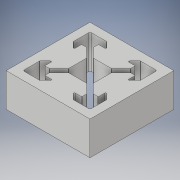
# Autodesk Inventor part: StepperMount
Saved by Autodesk Inventor 2019.4 (Build 234330000, 330)
## iProperties
Created: 2020-12-22
Part Number: StepperMount
Material: Generic
Document SubType Name: Modeling
Designer: Jorian Brusind
Density: 1 g/cm^3
Appearance: Default
Author: Jorian Brusind
Autodesk Inventor part; units mm, degrees
ref_plane "YZ Plane" through (0, 0, 0) normal (1, 0, 0) x (0, 1, 0)
ref_plane "XZ Plane" through (0, 0, 0) normal (0, 1, 0) x (-1, 0, 0)
ref_plane "XY Plane" through (0, 0, 0) normal (0, 0, 1) x (1, 0, 0)
sketch "2020 profile" plane through (0, 0, 0) normal (0, 0, 1) x (1, 0, 0)
  line L0 (8.75, -15.1376) -> (8.75, -9.8624)
  line L1 (2.5, -7.4482) -> (2.5, -3)
  line L2 (4.0732, -9.0732) -> (2.5366, -7.5366)
  line L3 (4.5, -7.125) -> (4.5, -8.8964)
  line L4 (5.8876, -7) -> (4.625, -7)
  line L5 (7, -4.625) -> (7, -5.8876)
  line L6 (7.0366, -5.976) -> (9.774, -8.7134)
  line L7 (8.8964, -4.5) -> (7.125, -4.5)
  line L8 (7.5366, -2.5366) -> (9.0732, -4.0732)
  line L9 (3, -2.5) -> (7.4482, -2.5)
  line L10 (17.5518, -2.5) -> (22, -2.5)
  arc A0 (22.5, -3) -> (22, -2.5) centre (22, -3) ccw
  line L11 (22.5, -3) -> (22.5, -7.4482)
  line L12 (22.4634, -7.5366) -> (20.9268, -9.0732)
  line L13 (20.5, -8.8964) -> (20.5, -7.125)
  line L14 (20.375, -7) -> (19.1124, -7)
  line L15 (18, -5.8876) -> (18, -4.625)
  line L16 (17.875, -4.5) -> (16.1036, -4.5)
  line L17 (15.226, -8.7134) -> (17.9634, -5.976)
  line L18 (19.024, -7.0366) -> (16.2866, -9.774)
  line L19 (16.25, -9.8624) -> (16.25, -15.1376)
  line L20 (16.2866, -15.226) -> (19.024, -17.9634)
  line L21 (19.1124, -18) -> (20.375, -18)
  arc A1 (19.024, -17.9634) -> (19.1124, -18) centre (19.1124, -17.875) ccw
  arc A2 (20.375, -18) -> (20.5, -17.875) centre (20.375, -17.875) ccw
  line L22 (20.5, -17.875) -> (20.5, -16.1036)
  arc A3 (20.9268, -15.9268) -> (20.5, -16.1036) centre (20.75, -16.1036) ccw
  line L23 (20.9268, -15.9268) -> (22.4634, -17.4634)
  arc A4 (22.5, -17.5518) -> (22.4634, -17.4634) centre (22.375, -17.5518) ccw
  line L24 (22.5, -17.5518) -> (22.5, -22)
  line L25 (22, -22.5) -> (17.5518, -22.5)
  line L26 (17.4634, -22.4634) -> (15.9268, -20.9268)
  arc A5 (16.1036, -20.5) -> (15.9268, -20.9268) centre (16.1036, -20.75) ccw
  line L27 (16.1036, -20.5) -> (17.875, -20.5)
  arc A6 (17.875, -20.5) -> (18, -20.375) centre (17.875, -20.375) ccw
  line L28 (18, -20.375) -> (18, -19.1124)
  arc A7 (18, -19.1124) -> (17.9634, -19.024) centre (17.875, -19.1124) ccw
  line L29 (17.9634, -19.024) -> (15.226, -16.2866)
  arc A8 (15.226, -16.2866) -> (15.1376, -16.25) centre (15.1376, -16.375) ccw
  line L30 (15.1376, -16.25) -> (9.8624, -16.25)
  arc A9 (9.8624, -16.25) -> (9.774, -16.2866) centre (9.8624, -16.375) ccw
  line L31 (9.774, -16.2866) -> (7.0366, -19.024)
  circle A10 centre (12.5, -12.5) radius 2
  line L32 (7.125, -20.5) -> (8.8964, -20.5)
  line L33 (9.0732, -20.9268) -> (7.5366, -22.4634)
  arc A11 (9.0732, -20.9268) -> (8.8964, -20.5) centre (8.8964, -20.75) ccw
  line L34 (7.4482, -22.5) -> (3, -22.5)
  arc A12 (7.4482, -22.5) -> (7.5366, -22.4634) centre (7.4482, -22.375) ccw
  arc A13 (7, -20.375) -> (7.125, -20.5) centre (7.125, -20.375) ccw
  line L35 (7, -19.1124) -> (7, -20.375)
  arc A14 (7.0366, -19.024) -> (7, -19.1124) centre (7.125, -19.1124) ccw
  arc A15 (2.5, -22) -> (3, -22.5) centre (3, -22) ccw
  line L36 (2.5, -22) -> (2.5, -17.5518)
  arc A16 (2.5366, -17.4634) -> (2.5, -17.5518) centre (2.625, -17.5518) ccw
  line L37 (2.5366, -17.4634) -> (4.0732, -15.9268)
  arc A17 (4.5, -16.1036) -> (4.0732, -15.9268) centre (4.25, -16.1036) ccw
  line L38 (4.5, -16.1036) -> (4.5, -17.875)
  arc A18 (4.5, -17.875) -> (4.625, -18) centre (4.625, -17.875) ccw
  line L39 (4.625, -18) -> (5.8876, -18)
  line L40 (5.976, -17.9634) -> (8.7134, -15.226)
  arc A19 (5.8876, -18) -> (5.976, -17.9634) centre (5.8876, -17.875) ccw
  arc A20 (8.75, -9.8624) -> (8.7134, -9.774) centre (8.625, -9.8624) ccw
  line L41 (8.7134, -9.774) -> (5.976, -7.0366)
  arc A21 (4.0732, -9.0732) -> (4.5, -8.8964) centre (4.25, -8.8964) ccw
  arc A22 (2.5, -7.4482) -> (2.5366, -7.5366) centre (2.625, -7.4482) ccw
  arc A23 (3, -2.5) -> (2.5, -3) centre (3, -3) ccw
  arc A24 (8.8964, -4.5) -> (9.0732, -4.0732) centre (8.8964, -4.25) ccw
  arc A25 (7.125, -4.5) -> (7, -4.625) centre (7.125, -4.625) ccw
  arc A26 (7.5366, -2.5366) -> (7.4482, -2.5) centre (7.4482, -2.625) ccw
  arc A27 (7, -5.8876) -> (7.0366, -5.976) centre (7.125, -5.8876) ccw
  arc A28 (9.774, -8.7134) -> (9.8624, -8.75) centre (9.8624, -8.625) ccw
  line L42 (9.8624, -8.75) -> (15.1376, -8.75)
  line L43 (15.9268, -4.0732) -> (17.4634, -2.5366)
  arc A29 (17.5518, -2.5) -> (17.4634, -2.5366) centre (17.5518, -2.625) ccw
  arc A30 (15.9268, -4.0732) -> (16.1036, -4.5) centre (16.1036, -4.25) ccw
  arc A31 (20.5, -8.8964) -> (20.9268, -9.0732) centre (20.75, -8.8964) ccw
  arc A32 (22, -22.5) -> (22.5, -22) centre (22, -22) ccw
  point P0 (12.1463, -12.8552)
sketch "2020 Tslot Extrusion" plane through (0, 0, 0) normal (0, 0, 1) x (1, 0, 0)
  line L0 (8.75, -15.1376) -> (8.75, -9.8624)
  line L1 (2.5, -7.4482) -> (2.5, -3)
  line L2 (4.0732, -9.0732) -> (2.5366, -7.5366)
  line L3 (4.5, -7.125) -> (4.5, -8.8964)
  line L4 (5.8876, -7) -> (4.625, -7)
  line L5 (7, -4.625) -> (7, -5.8876)
  line L6 (7.0366, -5.976) -> (9.774, -8.7134)
  line L7 (8.8964, -4.5) -> (7.125, -4.5)
  line L8 (7.5366, -2.5366) -> (9.0732, -4.0732)
  line L9 (3, -2.5) -> (7.4482, -2.5)
  line L10 (17.5518, -2.5) -> (22, -2.5)
  arc A0 (22.5, -3) -> (22, -2.5) centre (22, -3) ccw
  line L11 (22.5, -3) -> (22.5, -7.4482)
  line L12 (22.4634, -7.5366) -> (20.9268, -9.0732)
  line L13 (20.5, -8.8964) -> (20.5, -7.125)
  line L14 (20.375, -7) -> (19.1124, -7)
  line L15 (18, -5.8876) -> (18, -4.625)
  line L16 (17.875, -4.5) -> (16.1036, -4.5)
  line L17 (15.226, -8.7134) -> (17.9634, -5.976)
  line L18 (19.024, -7.0366) -> (16.2866, -9.774)
  line L19 (16.25, -9.8624) -> (16.25, -15.1376)
  line L20 (16.2866, -15.226) -> (19.024, -17.9634)
  line L21 (19.1124, -18) -> (20.375, -18)
  arc A1 (19.024, -17.9634) -> (19.1124, -18) centre (19.1124, -17.875) ccw
  arc A2 (20.375, -18) -> (20.5, -17.875) centre (20.375, -17.875) ccw
  line L22 (20.5, -17.875) -> (20.5, -16.1036)
  arc A3 (20.9268, -15.9268) -> (20.5, -16.1036) centre (20.75, -16.1036) ccw
  line L23 (20.9268, -15.9268) -> (22.4634, -17.4634)
  arc A4 (22.5, -17.5518) -> (22.4634, -17.4634) centre (22.375, -17.5518) ccw
  line L24 (22.5, -17.5518) -> (22.5, -22)
  line L25 (22, -22.5) -> (17.5518, -22.5)
  line L26 (17.4634, -22.4634) -> (15.9268, -20.9268)
  arc A5 (16.1036, -20.5) -> (15.9268, -20.9268) centre (16.1036, -20.75) ccw
  line L27 (16.1036, -20.5) -> (17.875, -20.5)
  arc A6 (17.875, -20.5) -> (18, -20.375) centre (17.875, -20.375) ccw
  line L28 (18, -20.375) -> (18, -19.1124)
  arc A7 (18, -19.1124) -> (17.9634, -19.024) centre (17.875, -19.1124) ccw
  line L29 (17.9634, -19.024) -> (15.226, -16.2866)
  arc A8 (15.226, -16.2866) -> (15.1376, -16.25) centre (15.1376, -16.375) ccw
  line L30 (15.1376, -16.25) -> (9.8624, -16.25)
  arc A9 (9.8624, -16.25) -> (9.774, -16.2866) centre (9.8624, -16.375) ccw
  line L31 (9.774, -16.2866) -> (7.0366, -19.024)
  circle A10 centre (12.5, -12.5) radius 2
  line L32 (7.125, -20.5) -> (8.8964, -20.5)
  line L33 (9.0732, -20.9268) -> (7.5366, -22.4634)
  arc A11 (9.0732, -20.9268) -> (8.8964, -20.5) centre (8.8964, -20.75) ccw
  line L34 (7.4482, -22.5) -> (3, -22.5)
  arc A12 (7.4482, -22.5) -> (7.5366, -22.4634) centre (7.4482, -22.375) ccw
  arc A13 (7, -20.375) -> (7.125, -20.5) centre (7.125, -20.375) ccw
  line L35 (7, -19.1124) -> (7, -20.375)
  arc A14 (7.0366, -19.024) -> (7, -19.1124) centre (7.125, -19.1124) ccw
  arc A15 (2.5, -22) -> (3, -22.5) centre (3, -22) ccw
  line L36 (2.5, -22) -> (2.5, -17.5518)
  arc A16 (2.5366, -17.4634) -> (2.5, -17.5518) centre (2.625, -17.5518) ccw
  line L37 (2.5366, -17.4634) -> (4.0732, -15.9268)
  arc A17 (4.5, -16.1036) -> (4.0732, -15.9268) centre (4.25, -16.1036) ccw
  line L38 (4.5, -16.1036) -> (4.5, -17.875)
  arc A18 (4.5, -17.875) -> (4.625, -18) centre (4.625, -17.875) ccw
  line L39 (4.625, -18) -> (5.8876, -18)
  line L40 (5.976, -17.9634) -> (8.7134, -15.226)
  arc A19 (5.8876, -18) -> (5.976, -17.9634) centre (5.8876, -17.875) ccw
  arc A20 (8.75, -9.8624) -> (8.7134, -9.774) centre (8.625, -9.8624) ccw
  line L41 (8.7134, -9.774) -> (5.976, -7.0366)
  arc A21 (4.0732, -9.0732) -> (4.5, -8.8964) centre (4.25, -8.8964) ccw
  arc A22 (2.5, -7.4482) -> (2.5366, -7.5366) centre (2.625, -7.4482) ccw
  arc A23 (3, -2.5) -> (2.5, -3) centre (3, -3) ccw
  arc A24 (8.8964, -4.5) -> (9.0732, -4.0732) centre (8.8964, -4.25) ccw
  arc A25 (7.125, -4.5) -> (7, -4.625) centre (7.125, -4.625) ccw
  arc A26 (7.5366, -2.5366) -> (7.4482, -2.5) centre (7.4482, -2.625) ccw
  arc A27 (7, -5.8876) -> (7.0366, -5.976) centre (7.125, -5.8876) ccw
  arc A28 (9.774, -8.7134) -> (9.8624, -8.75) centre (9.8624, -8.625) ccw
  line L42 (9.8624, -8.75) -> (15.1376, -8.75)
  line L43 (15.9268, -4.0732) -> (17.4634, -2.5366)
  arc A29 (17.5518, -2.5) -> (17.4634, -2.5366) centre (17.5518, -2.625) ccw
  arc A30 (15.9268, -4.0732) -> (16.1036, -4.5) centre (16.1036, -4.25) ccw
  arc A31 (20.5, -8.8964) -> (20.9268, -9.0732) centre (20.75, -8.8964) ccw
  arc A32 (22, -22.5) -> (22.5, -22) centre (22, -22) ccw
  arc A33 (18, -4.625) -> (17.875, -4.5) centre (17.875, -4.625) ccw
  arc A34 (17.9634, -5.976) -> (18, -5.8876) centre (17.875, -5.8876) ccw
  arc A35 (22.5, -3) -> (22, -2.5) centre (22, -3) ccw
  arc A36 (17.5518, -2.5) -> (17.4634, -2.5366) centre (17.5518, -2.625) ccw
  arc A37 (22.4634, -7.5366) -> (22.5, -7.4482) centre (22.375, -7.4482) ccw
  arc A38 (20.5, -8.8964) -> (20.9268, -9.0732) centre (20.75, -8.8964) ccw
  arc A39 (8.8964, -4.5) -> (9.0732, -4.0732) centre (8.8964, -4.25) ccw
  arc A40 (3, -2.5) -> (2.5, -3) centre (3, -3) ccw
  arc A41 (7.5366, -2.5366) -> (7.4482, -2.5) centre (7.4482, -2.625) ccw
  arc A42 (7.125, -4.5) -> (7, -4.625) centre (7.125, -4.625) ccw
  arc A43 (7, -5.8876) -> (7.0366, -5.976) centre (7.125, -5.8876) ccw
  arc A44 (9.774, -8.7134) -> (9.8624, -8.75) centre (9.8624, -8.625) ccw
  arc A45 (15.1376, -8.75) -> (15.226, -8.7134) centre (15.1376, -8.625) ccw
  arc A46 (4.625, -7) -> (4.5, -7.125) centre (4.625, -7.125) ccw
  arc A47 (4.0732, -9.0732) -> (4.5, -8.8964) centre (4.25, -8.8964) ccw
  arc A48 (5.976, -7.0366) -> (5.8876, -7) centre (5.8876, -7.125) ccw
  arc A49 (20.5, -7.125) -> (20.375, -7) centre (20.375, -7.125) ccw
  arc A50 (19.1124, -7) -> (19.024, -7.0366) centre (19.1124, -7.125) ccw
  arc A51 (16.2866, -9.774) -> (16.25, -9.8624) centre (16.375, -9.8624) ccw
  arc A52 (16.25, -15.1376) -> (16.2866, -15.226) centre (16.375, -15.1376) ccw
  arc A53 (8.7134, -15.226) -> (8.75, -15.1376) centre (8.625, -15.1376) ccw
  arc A54 (17.4634, -22.4634) -> (17.5518, -22.5) centre (17.5518, -22.375) ccw
  line L44 (5.5, -8.8964) -> (5.5, -8)
  line L45 (5.5, -8) -> (5.5251, -8)
  line L46 (5.5251, -8) -> (7.75, -10.2249)
  line L47 (7.75, -10.2249) -> (7.75, -14.7751)
  line L48 (7.75, -14.7751) -> (5.5251, -17)
  line L49 (5.5251, -17) -> (5.5, -17)
  line L50 (5.5, -17) -> (5.5, -16.1036)
  arc A55 (5.5, -16.1036) -> (3.3661, -15.2197) centre (4.25, -16.1036) ccw
  line L51 (3.3661, -15.2197) -> (1.8295, -16.7563)
  arc A56 (1.8295, -16.7563) -> (1.5, -17.5518) centre (2.625, -17.5518) ccw
  line L52 (1.5, -17.5518) -> (1.5, -22)
  arc A57 (1.5, -22) -> (3, -23.5) centre (3, -22) ccw
  line L53 (3, -23.5) -> (7.4482, -23.5)
  arc A58 (7.4482, -23.5) -> (8.2437, -23.1705) centre (7.4482, -22.375) ccw
  line L54 (8.2437, -23.1705) -> (9.7803, -21.6339)
  arc A59 (9.7803, -21.6339) -> (8.8964, -19.5) centre (8.8964, -20.75) ccw
  line L55 (8.8964, -19.5) -> (8, -19.5)
  line L56 (8, -19.5) -> (8, -19.4749)
  line L57 (8, -19.4749) -> (10.2249, -17.25)
  line L58 (10.2249, -17.25) -> (14.7751, -17.25)
  line L59 (14.7751, -17.25) -> (17, -19.4749)
  line L60 (17, -19.4749) -> (17, -19.5)
  line L61 (17, -19.5) -> (16.1036, -19.5)
  arc A60 (16.1036, -19.5) -> (15.2197, -21.6339) centre (16.1036, -20.75) ccw
  line L62 (15.2197, -21.6339) -> (16.7563, -23.1705)
  arc A61 (16.7563, -23.1705) -> (17.5518, -23.5) centre (17.5518, -22.375) ccw
  line L63 (17.5518, -23.5) -> (22, -23.5)
  arc A62 (22, -23.5) -> (23.5, -22) centre (22, -22) ccw
  line L64 (23.5, -22) -> (23.5, -17.5518)
  arc A63 (23.5, -17.5518) -> (23.1705, -16.7563) centre (22.375, -17.5518) ccw
  line L65 (23.1705, -16.7563) -> (21.6339, -15.2197)
  arc A64 (21.6339, -15.2197) -> (19.5, -16.1036) centre (20.75, -16.1036) ccw
  line L66 (19.5, -16.1036) -> (19.5, -17)
  line L67 (19.5, -17) -> (19.4749, -17)
  line L68 (19.4749, -17) -> (17.25, -14.7751)
  line L69 (17.25, -14.7751) -> (17.25, -10.2249)
  line L70 (17.25, -10.2249) -> (19.4749, -8)
  line L71 (19.4749, -8) -> (19.5, -8)
  line L72 (19.5, -8) -> (19.5, -8.8964)
  line L73 (9.8624, -7.75) -> (14.7751, -7.75)
  line L74 (14.7751, -7.75) -> (17, -5.5251)
  line L75 (17, -5.5251) -> (17, -5.5)
  line L76 (17, -5.5) -> (16.1036, -5.5)
  arc A65 (15.2197, -3.3661) -> (16.1036, -5.5) centre (16.1036, -4.25) ccw
  line L77 (15.2197, -3.3661) -> (16.7563, -1.8295)
  line L78 (17.5518, -1.5) -> (22, -1.5)
  arc A66 (17.5518, -1.5) -> (16.7563, -1.8295) centre (17.5518, -2.625) ccw
  line L79 (21.5, -3) -> (21.5, -7.0858)
  line L80 (21.5, -7.0858) -> (20.2197, -8.3661)
  point P0 (12.3493, -11.8573)
  dimension "d10" = 1
  dimension "d11" = 1
  dimension "d12" = 1
  dimension "d13" = 1
  dimension "d14" = 1
  measures "d10" distance between parallel lines of L0 L47
  measures "d11" distance between parallel lines of L42 L73
  measures "d12" distance between parallel lines of L10 L78
  measures "d13" radial gap between concentric circles of A29 A66
  measures "d14" distance between parallel lines of L11 L79
sketch "Sketch1" plane through (0, 0, 0) normal (0, 1, 0) x (-1, 0, 0)
  line L0 (0, 0) -> (25, 0)
  line L1 (25, 0) -> (25, -25)
  line L2 (25, -25) -> (0, -25)
  line L3 (0, -25) -> (0, 0)
  dimension "d0" = 25
  dimension "d1" = 25
  constraints: 8 end point, 2 parallel, 1 horizontal, 1 perpendicular
  measures "d0" distance of L1.end L2.end
  measures "d1" distance of L0.end L1.end
extrude "Extrusion1" add sketch "Sketch1" along normal blind 10
sketch "Sketch2" plane through (0, 10, 0) normal (0, 1, 0) x (1, 0, 0)
  line L0 (8.75, -15.1376) -> (8.75, -9.8624)
  line L1 (2.5, -7.4482) -> (2.5, -3)
  line L2 (4.0732, -9.0732) -> (2.5366, -7.5366)
  line L3 (4.5, -7.125) -> (4.5, -8.8964)
  line L4 (5.8876, -7) -> (4.625, -7)
  line L5 (7, -4.625) -> (7, -5.8876)
  line L6 (7.0366, -5.976) -> (9.774, -8.7134)
  line L7 (8.8964, -4.5) -> (7.125, -4.5)
  line L8 (7.5366, -2.5366) -> (9.0732, -4.0732)
  line L9 (3, -2.5) -> (7.4482, -2.5)
  line L10 (17.5518, -2.5) -> (22, -2.5)
  arc A0 (22.5, -3) -> (22, -2.5) centre (22, -3) ccw
  line L11 (22.5, -3) -> (22.5, -7.4482)
  line L12 (22.4634, -7.5366) -> (20.9268, -9.0732)
  line L13 (20.5, -8.8964) -> (20.5, -7.125)
  line L14 (20.375, -7) -> (19.1124, -7)
  line L15 (18, -5.8876) -> (18, -4.625)
  line L16 (17.875, -4.5) -> (16.1036, -4.5)
  line L17 (15.226, -8.7134) -> (17.9634, -5.976)
  line L18 (19.024, -7.0366) -> (16.2866, -9.774)
  line L19 (16.25, -9.8624) -> (16.25, -15.1376)
  line L20 (16.2866, -15.226) -> (19.024, -17.9634)
  line L21 (19.1124, -18) -> (20.375, -18)
  arc A1 (19.024, -17.9634) -> (19.1124, -18) centre (19.1124, -17.875) ccw
  arc A2 (20.375, -18) -> (20.5, -17.875) centre (20.375, -17.875) ccw
  line L22 (20.5, -17.875) -> (20.5, -16.1036)
  arc A3 (20.9268, -15.9268) -> (20.5, -16.1036) centre (20.75, -16.1036) ccw
  line L23 (20.9268, -15.9268) -> (22.4634, -17.4634)
  arc A4 (22.5, -17.5518) -> (22.4634, -17.4634) centre (22.375, -17.5518) ccw
  line L24 (22.5, -17.5518) -> (22.5, -22)
  line L25 (22, -22.5) -> (17.5518, -22.5)
  line L26 (17.4634, -22.4634) -> (15.9268, -20.9268)
  arc A5 (16.1036, -20.5) -> (15.9268, -20.9268) centre (16.1036, -20.75) ccw
  line L27 (16.1036, -20.5) -> (17.875, -20.5)
  arc A6 (17.875, -20.5) -> (18, -20.375) centre (17.875, -20.375) ccw
  line L28 (18, -20.375) -> (18, -19.1124)
  arc A7 (18, -19.1124) -> (17.9634, -19.024) centre (17.875, -19.1124) ccw
  line L29 (17.9634, -19.024) -> (15.226, -16.2866)
  arc A8 (15.226, -16.2866) -> (15.1376, -16.25) centre (15.1376, -16.375) ccw
  line L30 (15.1376, -16.25) -> (9.8624, -16.25)
  arc A9 (9.8624, -16.25) -> (9.774, -16.2866) centre (9.8624, -16.375) ccw
  line L31 (9.774, -16.2866) -> (7.0366, -19.024)
  circle A10 centre (12.5, -12.5) radius 2
  line L32 (7.125, -20.5) -> (8.8964, -20.5)
  line L33 (9.0732, -20.9268) -> (7.5366, -22.4634)
  arc A11 (9.0732, -20.9268) -> (8.8964, -20.5) centre (8.8964, -20.75) ccw
  line L34 (7.4482, -22.5) -> (3, -22.5)
  arc A12 (7.4482, -22.5) -> (7.5366, -22.4634) centre (7.4482, -22.375) ccw
  arc A13 (7, -20.375) -> (7.125, -20.5) centre (7.125, -20.375) ccw
  line L35 (7, -19.1124) -> (7, -20.375)
  arc A14 (7.0366, -19.024) -> (7, -19.1124) centre (7.125, -19.1124) ccw
  arc A15 (2.5, -22) -> (3, -22.5) centre (3, -22) ccw
  line L36 (2.5, -22) -> (2.5, -17.5518)
  arc A16 (2.5366, -17.4634) -> (2.5, -17.5518) centre (2.625, -17.5518) ccw
  line L37 (2.5366, -17.4634) -> (4.0732, -15.9268)
  arc A17 (4.5, -16.1036) -> (4.0732, -15.9268) centre (4.25, -16.1036) ccw
  line L38 (4.5, -16.1036) -> (4.5, -17.875)
  arc A18 (4.5, -17.875) -> (4.625, -18) centre (4.625, -17.875) ccw
  line L39 (4.625, -18) -> (5.8876, -18)
  line L40 (5.976, -17.9634) -> (8.7134, -15.226)
  arc A19 (5.8876, -18) -> (5.976, -17.9634) centre (5.8876, -17.875) ccw
  arc A20 (8.75, -9.8624) -> (8.7134, -9.774) centre (8.625, -9.8624) ccw
  line L41 (8.7134, -9.774) -> (5.976, -7.0366)
  arc A21 (4.0732, -9.0732) -> (4.5, -8.8964) centre (4.25, -8.8964) ccw
  arc A22 (2.5, -7.4482) -> (2.5366, -7.5366) centre (2.625, -7.4482) ccw
  arc A23 (3, -2.5) -> (2.5, -3) centre (3, -3) ccw
  arc A24 (8.8964, -4.5) -> (9.0732, -4.0732) centre (8.8964, -4.25) ccw
  arc A25 (7.125, -4.5) -> (7, -4.625) centre (7.125, -4.625) ccw
  arc A26 (7.5366, -2.5366) -> (7.4482, -2.5) centre (7.4482, -2.625) ccw
  arc A27 (7, -5.8876) -> (7.0366, -5.976) centre (7.125, -5.8876) ccw
  arc A28 (9.774, -8.7134) -> (9.8624, -8.75) centre (9.8624, -8.625) ccw
  line L42 (9.8624, -8.75) -> (15.1376, -8.75)
  line L43 (15.9268, -4.0732) -> (17.4634, -2.5366)
  arc A29 (17.5518, -2.5) -> (17.4634, -2.5366) centre (17.5518, -2.625) ccw
  arc A30 (15.9268, -4.0732) -> (16.1036, -4.5) centre (16.1036, -4.25) ccw
  arc A31 (20.5, -8.8964) -> (20.9268, -9.0732) centre (20.75, -8.8964) ccw
  arc A32 (22, -22.5) -> (22.5, -22) centre (22, -22) ccw
  arc A33 (18, -4.625) -> (17.875, -4.5) centre (17.875, -4.625) ccw
  arc A34 (17.9634, -5.976) -> (18, -5.8876) centre (17.875, -5.8876) ccw
  arc A35 (22.5, -3) -> (22, -2.5) centre (22, -3) ccw
  arc A36 (17.5518, -2.5) -> (17.4634, -2.5366) centre (17.5518, -2.625) ccw
  arc A37 (22.4634, -7.5366) -> (22.5, -7.4482) centre (22.375, -7.4482) ccw
  arc A38 (20.5, -8.8964) -> (20.9268, -9.0732) centre (20.75, -8.8964) ccw
  arc A39 (8.8964, -4.5) -> (9.0732, -4.0732) centre (8.8964, -4.25) ccw
  arc A40 (3, -2.5) -> (2.5, -3) centre (3, -3) ccw
  arc A41 (7.5366, -2.5366) -> (7.4482, -2.5) centre (7.4482, -2.625) ccw
  arc A42 (7.125, -4.5) -> (7, -4.625) centre (7.125, -4.625) ccw
  arc A43 (7, -5.8876) -> (7.0366, -5.976) centre (7.125, -5.8876) ccw
  arc A44 (9.774, -8.7134) -> (9.8624, -8.75) centre (9.8624, -8.625) ccw
  arc A45 (15.1376, -8.75) -> (15.226, -8.7134) centre (15.1376, -8.625) ccw
  arc A46 (4.625, -7) -> (4.5, -7.125) centre (4.625, -7.125) ccw
  arc A47 (4.0732, -9.0732) -> (4.5, -8.8964) centre (4.25, -8.8964) ccw
  arc A48 (5.976, -7.0366) -> (5.8876, -7) centre (5.8876, -7.125) ccw
  arc A49 (20.5, -7.125) -> (20.375, -7) centre (20.375, -7.125) ccw
  arc A50 (19.1124, -7) -> (19.024, -7.0366) centre (19.1124, -7.125) ccw
  arc A51 (16.2866, -9.774) -> (16.25, -9.8624) centre (16.375, -9.8624) ccw
  arc A52 (16.25, -15.1376) -> (16.2866, -15.226) centre (16.375, -15.1376) ccw
  arc A53 (8.7134, -15.226) -> (8.75, -15.1376) centre (8.625, -15.1376) ccw
  arc A54 (17.4634, -22.4634) -> (17.5518, -22.5) centre (17.5518, -22.375) ccw
  line L44 (5.5, -8.8964) -> (5.5, -8)
  line L45 (5.5, -8) -> (5.5251, -8)
  line L46 (5.5251, -8) -> (7.75, -10.2249)
  line L47 (7.75, -10.2249) -> (7.75, -14.7751)
  line L48 (7.75, -14.7751) -> (5.5251, -17)
  line L49 (5.5251, -17) -> (5.5, -17)
  line L50 (5.5, -17) -> (5.5, -16.1036)
  arc A55 (5.5, -16.1036) -> (3.3661, -15.2197) centre (4.25, -16.1036) ccw
  line L51 (3.3661, -15.2197) -> (1.8295, -16.7563)
  arc A56 (1.8295, -16.7563) -> (1.5, -17.5518) centre (2.625, -17.5518) ccw
  line L52 (1.5, -17.5518) -> (1.5, -22)
  arc A57 (1.5, -22) -> (3, -23.5) centre (3, -22) ccw
  line L53 (3, -23.5) -> (7.4482, -23.5)
  arc A58 (7.4482, -23.5) -> (8.2437, -23.1705) centre (7.4482, -22.375) ccw
  line L54 (8.2437, -23.1705) -> (9.7803, -21.6339)
  arc A59 (9.7803, -21.6339) -> (8.8964, -19.5) centre (8.8964, -20.75) ccw
  line L55 (8.8964, -19.5) -> (8, -19.5)
  line L56 (8, -19.5) -> (8, -19.4749)
  line L57 (8, -19.4749) -> (10.2249, -17.25)
  line L58 (10.2249, -17.25) -> (14.7751, -17.25)
  line L59 (14.7751, -17.25) -> (17, -19.4749)
  line L60 (17, -19.4749) -> (17, -19.5)
  line L61 (17, -19.5) -> (16.1036, -19.5)
  arc A60 (16.1036, -19.5) -> (15.2197, -21.6339) centre (16.1036, -20.75) ccw
  line L62 (15.2197, -21.6339) -> (16.7563, -23.1705)
  arc A61 (16.7563, -23.1705) -> (17.5518, -23.5) centre (17.5518, -22.375) ccw
  line L63 (17.5518, -23.5) -> (22, -23.5)
  arc A62 (22, -23.5) -> (23.5, -22) centre (22, -22) ccw
  line L64 (23.5, -22) -> (23.5, -17.5518)
  arc A63 (23.5, -17.5518) -> (23.1705, -16.7563) centre (22.375, -17.5518) ccw
  line L65 (23.1705, -16.7563) -> (21.6339, -15.2197)
  arc A64 (21.6339, -15.2197) -> (19.5, -16.1036) centre (20.75, -16.1036) ccw
  line L66 (19.5, -16.1036) -> (19.5, -17)
  line L67 (19.5, -17) -> (19.4749, -17)
  line L68 (19.4749, -17) -> (17.25, -14.7751)
  line L69 (17.25, -14.7751) -> (17.25, -10.2249)
  line L70 (17.25, -10.2249) -> (19.4749, -8)
  line L71 (19.4749, -8) -> (19.5, -8)
  line L72 (19.5, -8) -> (19.5, -8.8964)
  line L73 (9.8624, -7.75) -> (14.7751, -7.75)
  line L74 (14.7751, -7.75) -> (17, -5.5251)
  line L75 (17, -5.5251) -> (17, -5.5)
  line L76 (17, -5.5) -> (16.1036, -5.5)
  arc A65 (15.2197, -3.3661) -> (16.1036, -5.5) centre (16.1036, -4.25) ccw
  line L77 (15.2197, -3.3661) -> (16.7563, -1.8295)
  line L78 (17.5518, -1.5) -> (22, -1.5)
  arc A66 (17.5518, -1.5) -> (16.7563, -1.8295) centre (17.5518, -2.625) ccw
  line L79 (21.5, -3) -> (21.5, -7.0858)
  line L80 (21.5, -7.0858) -> (20.2197, -8.3661)
  point P0 (0, 0)
sketch "Sketch3" plane through (0, 10, 0) normal (0, 1, 0) x (1, 0, 0)
  line L0 (0, 25) -> (-25, 25) projected
  line L1 (-25, 25) -> (-25, 0) projected
  line L2 (-16.25, 9.8624) -> (-16.25, 15.1376)
  line L3 (-22.5, 17.5518) -> (-22.5, 22)
  line L4 (-20.9268, 15.9268) -> (-22.4634, 17.4634)
  line L5 (-20.5, 17.875) -> (-20.5, 16.1036)
  line L6 (-19.1124, 18) -> (-20.375, 18)
  line L7 (-18, 20.375) -> (-18, 19.1124)
  line L8 (-17.9634, 19.024) -> (-15.226, 16.2866)
  line L9 (-16.1036, 20.5) -> (-17.875, 20.5)
  line L10 (-17.4634, 22.4634) -> (-15.9268, 20.9268)
  line L11 (-22, 22.5) -> (-17.5518, 22.5)
  line L12 (-7.4482, 22.5) -> (-3, 22.5)
  arc A0 (-2.5, 22) -> (-3, 22.5) centre (-3, 22) ccw
  line L13 (-2.5, 22) -> (-2.5, 17.5518)
  line L14 (-2.5366, 17.4634) -> (-4.0732, 15.9268)
  line L15 (-4.5, 16.1036) -> (-4.5, 17.875)
  line L16 (-4.625, 18) -> (-5.8876, 18)
  line L17 (-7, 19.1124) -> (-7, 20.375)
  line L18 (-7.125, 20.5) -> (-8.8964, 20.5)
  line L19 (-9.774, 16.2866) -> (-7.0366, 19.024)
  line L20 (-5.976, 17.9634) -> (-8.7134, 15.226)
  line L21 (-8.75, 15.1376) -> (-8.75, 9.8624)
  line L22 (-8.7134, 9.774) -> (-5.976, 7.0366)
  line L23 (-5.8876, 7) -> (-4.625, 7)
  arc A1 (-5.976, 7.0366) -> (-5.8876, 7) centre (-5.8876, 7.125) ccw
  arc A2 (-4.625, 7) -> (-4.5, 7.125) centre (-4.625, 7.125) ccw
  line L24 (-4.5, 7.125) -> (-4.5, 8.8964)
  arc A3 (-4.0732, 9.0732) -> (-4.5, 8.8964) centre (-4.25, 8.8964) ccw
  line L25 (-4.0732, 9.0732) -> (-2.5366, 7.5366)
  arc A4 (-2.5, 7.4482) -> (-2.5366, 7.5366) centre (-2.625, 7.4482) ccw
  line L26 (-2.5, 7.4482) -> (-2.5, 3)
  line L27 (-3, 2.5) -> (-7.4482, 2.5)
  line L28 (-7.5366, 2.5366) -> (-9.0732, 4.0732)
  arc A5 (-8.8964, 4.5) -> (-9.0732, 4.0732) centre (-8.8964, 4.25) ccw
  line L29 (-8.8964, 4.5) -> (-7.125, 4.5)
  arc A6 (-7.125, 4.5) -> (-7, 4.625) centre (-7.125, 4.625) ccw
  line L30 (-7, 4.625) -> (-7, 5.8876)
  arc A7 (-7, 5.8876) -> (-7.0366, 5.976) centre (-7.125, 5.8876) ccw
  line L31 (-7.0366, 5.976) -> (-9.774, 8.7134)
  arc A8 (-9.774, 8.7134) -> (-9.8624, 8.75) centre (-9.8624, 8.625) ccw
  line L32 (-9.8624, 8.75) -> (-15.1376, 8.75)
  arc A9 (-15.1376, 8.75) -> (-15.226, 8.7134) centre (-15.1376, 8.625) ccw
  line L33 (-15.226, 8.7134) -> (-17.9634, 5.976)
  circle A10 centre (-12.5, 12.5) radius 2
  line L34 (-17.875, 4.5) -> (-16.1036, 4.5)
  line L35 (-15.9268, 4.0732) -> (-17.4634, 2.5366)
  arc A11 (-15.9268, 4.0732) -> (-16.1036, 4.5) centre (-16.1036, 4.25) ccw
  line L36 (-17.5518, 2.5) -> (-22, 2.5)
  arc A12 (-17.5518, 2.5) -> (-17.4634, 2.5366) centre (-17.5518, 2.625) ccw
  arc A13 (-18, 4.625) -> (-17.875, 4.5) centre (-17.875, 4.625) ccw
  line L37 (-18, 5.8876) -> (-18, 4.625)
  arc A14 (-17.9634, 5.976) -> (-18, 5.8876) centre (-17.875, 5.8876) ccw
  arc A15 (-22.5, 3) -> (-22, 2.5) centre (-22, 3) ccw
  line L38 (-22.5, 3) -> (-22.5, 7.4482)
  arc A16 (-22.4634, 7.5366) -> (-22.5, 7.4482) centre (-22.375, 7.4482) ccw
  line L39 (-22.4634, 7.5366) -> (-20.9268, 9.0732)
  arc A17 (-20.5, 8.8964) -> (-20.9268, 9.0732) centre (-20.75, 8.8964) ccw
  line L40 (-20.5, 8.8964) -> (-20.5, 7.125)
  arc A18 (-20.5, 7.125) -> (-20.375, 7) centre (-20.375, 7.125) ccw
  line L41 (-20.375, 7) -> (-19.1124, 7)
  line L42 (-19.024, 7.0366) -> (-16.2866, 9.774)
  arc A19 (-19.1124, 7) -> (-19.024, 7.0366) centre (-19.1124, 7.125) ccw
  arc A20 (-16.25, 15.1376) -> (-16.2866, 15.226) centre (-16.375, 15.1376) ccw
  line L43 (-16.2866, 15.226) -> (-19.024, 17.9634)
  arc A21 (-20.9268, 15.9268) -> (-20.5, 16.1036) centre (-20.75, 16.1036) ccw
  arc A22 (-22.5, 17.5518) -> (-22.4634, 17.4634) centre (-22.375, 17.5518) ccw
  arc A23 (-22, 22.5) -> (-22.5, 22) centre (-22, 22) ccw
  arc A24 (-16.1036, 20.5) -> (-15.9268, 20.9268) centre (-16.1036, 20.75) ccw
  arc A25 (-17.875, 20.5) -> (-18, 20.375) centre (-17.875, 20.375) ccw
  arc A26 (-17.4634, 22.4634) -> (-17.5518, 22.5) centre (-17.5518, 22.375) ccw
  arc A27 (-18, 19.1124) -> (-17.9634, 19.024) centre (-17.875, 19.1124) ccw
  arc A28 (-15.226, 16.2866) -> (-15.1376, 16.25) centre (-15.1376, 16.375) ccw
  line L44 (-15.1376, 16.25) -> (-9.8624, 16.25)
  line L45 (-9.0732, 20.9268) -> (-7.5366, 22.4634)
  arc A29 (-7.4482, 22.5) -> (-7.5366, 22.4634) centre (-7.4482, 22.375) ccw
  arc A30 (-9.0732, 20.9268) -> (-8.8964, 20.5) centre (-8.8964, 20.75) ccw
  arc A31 (-4.5, 16.1036) -> (-4.0732, 15.9268) centre (-4.25, 16.1036) ccw
  arc A32 (-3, 2.5) -> (-2.5, 3) centre (-3, 3) ccw
  arc A33 (-7, 20.375) -> (-7.125, 20.5) centre (-7.125, 20.375) ccw
  arc A34 (-7.0366, 19.024) -> (-7, 19.1124) centre (-7.125, 19.1124) ccw
  arc A35 (-2.5, 22) -> (-3, 22.5) centre (-3, 22) ccw
  arc A36 (-7.4482, 22.5) -> (-7.5366, 22.4634) centre (-7.4482, 22.375) ccw
  arc A37 (-2.5366, 17.4634) -> (-2.5, 17.5518) centre (-2.625, 17.5518) ccw
  arc A38 (-4.5, 16.1036) -> (-4.0732, 15.9268) centre (-4.25, 16.1036) ccw
  arc A39 (-16.1036, 20.5) -> (-15.9268, 20.9268) centre (-16.1036, 20.75) ccw
  arc A40 (-22, 22.5) -> (-22.5, 22) centre (-22, 22) ccw
  arc A41 (-17.4634, 22.4634) -> (-17.5518, 22.5) centre (-17.5518, 22.375) ccw
  arc A42 (-17.875, 20.5) -> (-18, 20.375) centre (-17.875, 20.375) ccw
  arc A43 (-18, 19.1124) -> (-17.9634, 19.024) centre (-17.875, 19.1124) ccw
  arc A44 (-15.226, 16.2866) -> (-15.1376, 16.25) centre (-15.1376, 16.375) ccw
  arc A45 (-9.8624, 16.25) -> (-9.774, 16.2866) centre (-9.8624, 16.375) ccw
  arc A46 (-20.375, 18) -> (-20.5, 17.875) centre (-20.375, 17.875) ccw
  arc A47 (-20.9268, 15.9268) -> (-20.5, 16.1036) centre (-20.75, 16.1036) ccw
  arc A48 (-19.024, 17.9634) -> (-19.1124, 18) centre (-19.1124, 17.875) ccw
  arc A49 (-4.5, 17.875) -> (-4.625, 18) centre (-4.625, 17.875) ccw
  arc A50 (-5.8876, 18) -> (-5.976, 17.9634) centre (-5.8876, 17.875) ccw
  arc A51 (-8.7134, 15.226) -> (-8.75, 15.1376) centre (-8.625, 15.1376) ccw
  arc A52 (-8.75, 9.8624) -> (-8.7134, 9.774) centre (-8.625, 9.8624) ccw
  arc A53 (-16.2866, 9.774) -> (-16.25, 9.8624) centre (-16.375, 9.8624) ccw
  arc A54 (-7.5366, 2.5366) -> (-7.4482, 2.5) centre (-7.4482, 2.625) ccw
  line L46 (-19.5, 16.1036) -> (-19.5, 17)
  line L47 (-19.5, 17) -> (-19.4749, 17)
  line L48 (-19.4749, 17) -> (-17.25, 14.7751)
  line L49 (-17.25, 14.7751) -> (-17.25, 10.2249)
  line L50 (-17.25, 10.2249) -> (-19.4749, 8)
  line L51 (-19.4749, 8) -> (-19.5, 8)
  line L52 (-19.5, 8) -> (-19.5, 8.8964)
  arc A55 (-19.5, 8.8964) -> (-21.6339, 9.7803) centre (-20.75, 8.8964) ccw
  line L53 (-21.6339, 9.7803) -> (-23.1705, 8.2437)
  arc A56 (-23.1705, 8.2437) -> (-23.5, 7.4482) centre (-22.375, 7.4482) ccw
  line L54 (-23.5, 7.4482) -> (-23.5, 3)
  arc A57 (-23.5, 3) -> (-22, 1.5) centre (-22, 3) ccw
  line L55 (-22, 1.5) -> (-17.5518, 1.5)
  arc A58 (-17.5518, 1.5) -> (-16.7563, 1.8295) centre (-17.5518, 2.625) ccw
  line L56 (-16.7563, 1.8295) -> (-15.2197, 3.3661)
  arc A59 (-15.2197, 3.3661) -> (-16.1036, 5.5) centre (-16.1036, 4.25) ccw
  line L57 (-16.1036, 5.5) -> (-17, 5.5)
  line L58 (-17, 5.5) -> (-17, 5.5251)
  line L59 (-17, 5.5251) -> (-14.7751, 7.75)
  line L60 (-14.7751, 7.75) -> (-10.2249, 7.75)
  line L61 (-10.2249, 7.75) -> (-8, 5.5251)
  line L62 (-8, 5.5251) -> (-8, 5.5)
  line L63 (-8, 5.5) -> (-8.8964, 5.5)
  arc A60 (-8.8964, 5.5) -> (-9.7803, 3.3661) centre (-8.8964, 4.25) ccw
  line L64 (-9.7803, 3.3661) -> (-8.2437, 1.8295)
  arc A61 (-8.2437, 1.8295) -> (-7.4482, 1.5) centre (-7.4482, 2.625) ccw
  line L65 (-7.4482, 1.5) -> (-3, 1.5)
  arc A62 (-3, 1.5) -> (-1.5, 3) centre (-3, 3) ccw
  line L66 (-1.5, 3) -> (-1.5, 7.4482)
  arc A63 (-1.5, 7.4482) -> (-1.8295, 8.2437) centre (-2.625, 7.4482) ccw
  line L67 (-1.8295, 8.2437) -> (-3.3661, 9.7803)
  arc A64 (-3.3661, 9.7803) -> (-5.5, 8.8964) centre (-4.25, 8.8964) ccw
  line L68 (-5.5, 8.8964) -> (-5.5, 8)
  line L69 (-5.5, 8) -> (-5.5251, 8)
  line L70 (-5.5251, 8) -> (-7.75, 10.2249)
  line L71 (-7.75, 10.2249) -> (-7.75, 14.7751)
  line L72 (-7.75, 14.7751) -> (-5.5251, 17)
  line L73 (-5.5251, 17) -> (-5.5, 17)
  line L74 (-5.5, 17) -> (-5.5, 16.1036)
  line L75 (-15.1376, 17.25) -> (-10.2249, 17.25)
  line L76 (-10.2249, 17.25) -> (-8, 19.4749)
  line L77 (-8, 19.4749) -> (-8, 19.5)
  line L78 (-8, 19.5) -> (-8.8964, 19.5)
  arc A65 (-9.7803, 21.6339) -> (-8.8964, 19.5) centre (-8.8964, 20.75) ccw
  line L79 (-9.7803, 21.6339) -> (-8.2437, 23.1705)
  line L80 (-7.4482, 23.5) -> (-3, 23.5)
  arc A66 (-7.4482, 23.5) -> (-8.2437, 23.1705) centre (-7.4482, 22.375) ccw
  line L81 (-3.5, 22) -> (-3.5, 17.9142)
  line L82 (-3.5, 17.9142) -> (-4.7803, 16.6339)
  point P0 (0, 0)
  dimension "d6" = 12.5
  dimension "d7" = 12.5
extrude "Extrusion2" cut sketch "Sketch3" against normal blind 10 contours L2 A20 L43 A48 L6 A46 L5 A21 L4 A22 L3 A23 L11 A26 L10 A24 L9 A25 L7 A27 L8 A28 L44 A45 L19 A34 L17 A33 L18 A30 L45 A29 L12 A0 L13 A37 L14 A31 L15 A49 L16 A50 L20 A51 L21 A52 L22 A1 L23 A2 L24 A3 L25 A4 L26 A32 L27 A54 L28 A5 L29 A6 L30 A7 L31 A8 L32 A9 L33 A14 L37 A13 L34 A11 L35 A12 L36 A15 L38 A16 L39 A17 L40 A18 L41 A19 L42 A53 | A10
body "Solid1"
